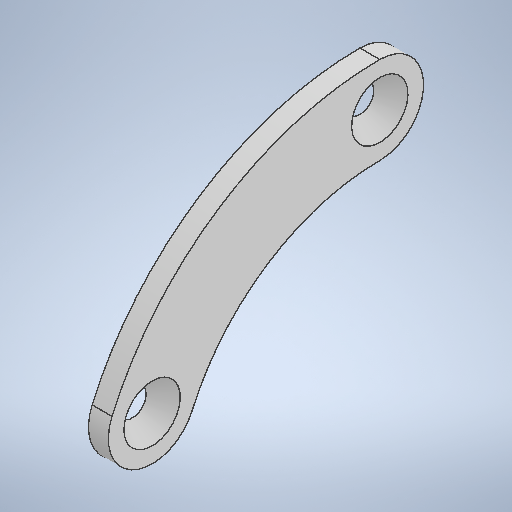
# Autodesk Inventor part: Mechanische_Anschlaege_Clip
Saved by Autodesk Inventor 2026.2 (Build 302298000, 298)
## iProperties
Created: 2026-03-24
Part Number: Mechanische_Anschlaege_Clip
Material: Generic
Document SubType Name: Modeling
Designer: Paco Ariel
Density: 1 g/cm^3
Appearance: Default
Author: Paco Ariel
Autodesk Inventor part; units mm, degrees
ref_plane "YZ Plane" through (0, 0, 0) normal (1, 0, 0) x (0, 1, 0)
ref_plane "XZ Plane" through (0, 0, 0) normal (0, 1, 0) x (-1, 0, 0)
ref_plane "XY Plane" through (0, 0, 0) normal (0, 0, 1) x (1, 0, 0)
sketch "Sketch1" plane through (0, 0, 0) normal (1, 0, 0) x (0, 1, 0)
  arc A0 (30.9, 0) -> (12.381, 28.3112) centre (0, 0) ccw
  arc A1 (44.1, 0) -> (17.6699, 40.4052) centre (0, 0) ccw
  line L0 (12.381, 28.3112) -> (17.6699, 40.4052)
  line L1 (30.9, 0) -> (44.1, 0) construction
  arc A2 (17.6699, 40.4052) -> (12.381, 28.3112) centre (15.0255, 34.3582) ccw
  arc A3 (30.9, 0) -> (44.1, 0) centre (37.5, 0) ccw
  circle A4 centre (15.0255, 34.3582) radius 2.1
  circle A5 centre (37.5, 0) radius 2.1
  dimension "d0" = 61.8
  dimension "d1" = 88.2
  dimension "d2" = 66.379
  dimension "d3" = 4.2
  dimension "d4" = 4.2
  constraints: 8 point on circle, 6 centre point, 4 coincident, 4 end point, 2 midpoint, 1 horizontal
  measures "d0" diameter of A0
  measures "d1" diameter of A1
  measures "d2" angle of L1 L0
  measures "d3" diameter of A4
  measures "d4" diameter of A5
extrude "Extrusion1" add sketch "Sketch1" along normal blind 3 contours A0 L0 A4 A1 A3 | A2 L0 A4
chamfer "Chamfer1" distance 2.15 distance2 3 2 edges at (3, 12.9255, 34.3582) (3, 35.4, 0) measured on face at (3, 38.069, 10.7229)
body "Solid1"
